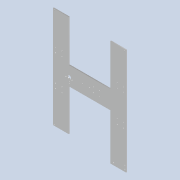
# Autodesk Inventor part: 0008-10-018 Suport Heated Bed
Saved by Autodesk Inventor 2020 (Build 240168000, 168)
## iProperties
Created: 2021-02-27
Part Number: 0008-10-018 Suport Heated Bed
Material: Aluminum 6061
Document SubType Name: Modeling
Designer: Iulian Bors
Density: 2.7 g/cm^3
Appearance: Aluminum - Flat
Mass: 812.917 g
Surface Area: 1617.85 cm^2
Volume: 301.08 cm^3
Description: SUport Pat
Author: Iulian Bors
Subject: 018
Autodesk Inventor part; units mm, degrees
ref_plane "YZ Plane" through (0, 0, 0) normal (1, 0, 0) x (0, 1, 0)
ref_plane "XZ Plane" through (0, 0, 0) normal (0, 1, 0) x (-1, 0, 0)
ref_plane "XY Plane" through (0, 0, 0) normal (0, 0, 1) x (1, 0, 0)
sketch "Sketch1" plane through (0, 0, 0) normal (0, 0, 1) x (1, 0, 0)
  line L0 (-158.5, 220) -> (158.5, 220)
  line L1 (158.5, 220) -> (158.5, -220)
  line L2 (158.5, -220) -> (-158.5, -220)
  line L3 (-158.5, -220) -> (-158.5, 220)
  line L4 (-153.5, 215) -> (153.5, 215) construction
  line L5 (153.5, 215) -> (153.5, -215) construction
  line L6 (153.5, -215) -> (-153.5, -215) construction
  line L7 (-153.5, -215) -> (-153.5, 215) construction
  circle A0 centre (-153.5, 215) radius 2
  circle A1 centre (153.5, 215) radius 2
  circle A2 centre (153.5, -215) radius 2
  circle A3 centre (-153.5, -215) radius 2
  point P0 (0, 0)
  point P1 (0, 220)
  point P2 (-158.5, 0)
  point P3 (0, 215)
  point P4 (-153.5, 0)
  dimension "d0" = 440
  dimension "d1" = 317
  dimension "d3" = 5
  dimension "d4" = 5
  dimension "d5" = 4
  constraints: 16 end point, 4 centre point, 4 coincident, 4 midpoint, 4 parallel, 3 equal radius, 2 horizontal, 2 horizontal alignment, 2 perpendicular, 2 vertical alignment
  measures "d0" distance of L2.end L0.start
  measures "d1" distance of L1.end L2.end
  measures "d3" distance between parallel lines of L3 L7
  measures "d4" distance between parallel lines of L0 L4
  measures "d5" diameter of A0
extrude "Extrusion1" add sketch "Sketch1" along normal blind 4
sketch "Sketch3" plane through (0, 0, 0) normal (0, 0, -1) x (-1, 0, 0)
  line L0 (90, -220) -> (-90, -220)
  line L1 (-90, -220) -> (-90, 220)
  line L2 (-90, 220) -> (90, 220)
  line L3 (90, 220) -> (90, -220)
  line L4 (158.5, -220) -> (-158.5, -220) projected
  line L5 (-158.5, 220) -> (158.5, 220) projected
  line L6 (90, -40) -> (-90, -40)
  line L7 (-90, -40) -> (-90, 40)
  line L8 (-90, 40) -> (90, 40)
  line L9 (90, 40) -> (90, -40)
  point P0 (0, 0)
  point P1 (0, -220)
  point P2 (-90, 0)
  dimension "d11" = 180
  dimension "d12" = 80
  constraints: 16 end point, 4 collinear, 4 parallel, 2 horizontal, 2 midpoint, 2 perpendicular, 1 horizontal alignment, 1 vertical alignment
  measures "d11" distance between parallel lines of L1 L3
  measures "d12" distance between parallel lines of L8 L6
extrude "Extrusion3" cut sketch "Sketch3" against normal through all contours L0 L1 L6 L3 | L8 L1 L2 L3
sketch "Sketch5" plane through (0, 0, 4) normal (0, 0, 1) x (1, 0, 0)
  line L0 (158.5, -240) -> (90, -240)
  line L1 (90, -240) -> (90, -220)
  line L2 (90, -220) -> (158.5, -220)
  line L3 (158.5, -220) -> (158.5, -240)
  line L4 (158.5, 220) -> (90, 220) projected
  line L5 (158.5, -220) -> (158.5, 220) projected
  line L6 (90, 220) -> (90, 40) projected
  circle A0 centre (153.5, -230) radius 2.5
  circle A1 centre (103.5, -230) radius 2.5
  line L7 (90, -220) -> (158.5, -220) projected
  point P0 (0, 0)
  point P1 (124.25, 201.6144)
  point P2 (124.25, -240)
  point P3 (90, -230)
  dimension "d21" = 20
  dimension "d22" = 5
  dimension "d24" = 50
  dimension "d34" = 5
  constraints: 8 end point, 3 collinear, 2 centre point, 2 horizontal alignment, 2 midpoint, 2 parallel, 1 equal radius, 1 horizontal, 1 perpendicular, 1 vertical alignment
  measures "d21" distance of L2.end L0.start
  measures "d22" diameter of A0
  measures "d24" distance of A1.centre A0.centre
  measures "d34" distance from line of A0.centre L3
extrude "Extrusion5" add sketch "Sketch5" against normal up to surface (4 mm away)
sketch "Sketch6" plane through (0, 0, 0) normal (0, 0, -1) x (-1, 0, 0)
  circle A0 centre (119.5, -78) radius 2.1
  circle A1 centre (147.5, -78) radius 2.1
  circle A2 centre (119.5, -57) radius 2.1
  circle A3 centre (147.5, -57) radius 2.1
  line L0 (152.5, -85) -> (142.5, -85)
  line L1 (142.5, -85) -> (142.5, -50)
  line L2 (142.5, -50) -> (152.5, -50)
  line L3 (152.5, -50) -> (152.5, -85)
  line L4 (137.5, -85) -> (129.5, -85)
  line L5 (129.5, -85) -> (129.5, -50)
  line L6 (129.5, -50) -> (137.5, -50)
  line L7 (137.5, -50) -> (137.5, -85)
  line L8 (124.5, -85) -> (114.5, -85)
  line L9 (114.5, -85) -> (114.5, -50)
  line L10 (114.5, -50) -> (124.5, -50)
  line L11 (124.5, -50) -> (124.5, -85)
  circle A4 centre (119.5, 57) radius 2.1
  circle A5 centre (147.5, 57) radius 2.1
  circle A6 centre (119.5, 78) radius 2.1
  circle A7 centre (147.5, 78) radius 2.1
  line L12 (152.5, 50) -> (142.5, 50)
  line L13 (142.5, 50) -> (142.5, 85)
  line L14 (142.5, 85) -> (152.5, 85)
  line L15 (152.5, 85) -> (152.5, 50)
  line L16 (137.5, 50) -> (129.5, 50)
  line L17 (129.5, 50) -> (129.5, 85)
  line L18 (129.5, 85) -> (137.5, 85)
  line L19 (137.5, 85) -> (137.5, 50)
  line L20 (124.5, 50) -> (114.5, 50)
  line L21 (114.5, 50) -> (114.5, 85)
  line L22 (114.5, 85) -> (124.5, 85)
  line L23 (124.5, 85) -> (124.5, 50)
  circle A8 centre (1, 0) radius 2.5
  circle A9 centre (30, 0) radius 2.5
  line L24 (10.5, -12) -> (30.5, -12)
  line L25 (30.5, -12) -> (30.5, -5)
  line L26 (30.5, -5) -> (10.5, -5)
  line L27 (10.5, -5) -> (10.5, -12)
  line L28 (-50, -15.5) -> (40, -15.5)
  line L29 (40, 15.5) -> (40, -15.5)
  line L30 (40, 15.5) -> (-50, 15.5)
  line L31 (-50, -15.5) -> (-50, 15.5)
  line L32 (30.5, 12) -> (10.5, 12)
  line L33 (10.5, 12) -> (10.5, 5)
  line L34 (10.5, 5) -> (30.5, 5)
  line L35 (30.5, 5) -> (30.5, 12)
  circle A10 centre (-16, -10.5) radius 3
  circle A11 centre (-44, -10.5) radius 3
  circle A12 centre (-44, 10.5) radius 3
  circle A13 centre (-16, 10.5) radius 3
  circle A14 centre (-119.5, -57) radius 2.1
  circle A15 centre (-147.5, -57) radius 2.1
  circle A16 centre (-119.5, -78) radius 2.1
  circle A17 centre (-147.5, -78) radius 2.1
  line L36 (-152.5, -50) -> (-142.5, -50)
  line L37 (-142.5, -50) -> (-142.5, -85)
  line L38 (-142.5, -85) -> (-152.5, -85)
  line L39 (-152.5, -85) -> (-152.5, -50)
  line L40 (-137.5, -50) -> (-129.5, -50)
  line L41 (-129.5, -50) -> (-129.5, -85)
  line L42 (-129.5, -85) -> (-137.5, -85)
  line L43 (-137.5, -85) -> (-137.5, -50)
  line L44 (-124.5, -50) -> (-114.5, -50)
  line L45 (-114.5, -50) -> (-114.5, -85)
  line L46 (-114.5, -85) -> (-124.5, -85)
  line L47 (-124.5, -85) -> (-124.5, -50)
  circle A18 centre (-147.5, 57) radius 2.1
  circle A19 centre (-119.5, 57) radius 2.1
  circle A20 centre (-147.5, 78) radius 2.1
  circle A21 centre (-119.5, 78) radius 2.1
  line L48 (-114.5, 50) -> (-124.5, 50)
  line L49 (-124.5, 50) -> (-124.5, 85)
  line L50 (-124.5, 85) -> (-114.5, 85)
  line L51 (-114.5, 85) -> (-114.5, 50)
  line L52 (-129.5, 50) -> (-137.5, 50)
  line L53 (-137.5, 50) -> (-137.5, 85)
  line L54 (-137.5, 85) -> (-129.5, 85)
  line L55 (-129.5, 85) -> (-129.5, 50)
  line L56 (-142.5, 50) -> (-152.5, 50)
  line L57 (-152.5, 50) -> (-152.5, 85)
  line L58 (-152.5, 85) -> (-142.5, 85)
  line L59 (-142.5, 85) -> (-142.5, 50)
  point P0 (0, 0)
  constraints: 120 end point, 30 horizontal, 30 vertical, 22 centre point, 104 other
hole "Hole1" at (-147.5, -78, 0) at (-119.5, -78, 0) at (-119.5, -57, 0) at (-147.5, -57, 0) at (-30, 0, 0) at (0, 0, 0) at (16, -10.5, 0) at (44, -10.5, 0) at (44, 10.5, 0) at (16, 10.5, 0) at (-119.5, 57, 0) at (-119.5, 78, 0) at (-147.5, 78, 0) at (-147.5, 57, 0) at (119.5, 57, 0) at (147.5, 57, 0) at (147.5, 78, 0) at (119.5, 78, 0) at (147.5, -78, 0) at (119.5, -78, 0) at (119.5, -57, 0) at (147.5, -57, 0) direction (0, 0, 1) diameter 5 end through all
sketch "Sketch7" plane through (0, 0, 0) normal (0, 0, -1) x (-1, 0, 0)
  line L0 (-60, -15.1293) -> (-60, -45.1293)
  line L1 (-71, -45.1293) -> (-60, -45.1293)
  line L2 (-71, -45.1293) -> (-71, -15.1293)
  line L3 (-71, -15.1293) -> (-60, -15.1293)
  circle A0 centre (88, -28) radius 2
  circle A1 centre (88, -20) radius 2
  line L4 (-90, -40) -> (90, -40) projected
  circle A2 centre (88, -5) radius 7.5
  circle A3 centre (76, -10) radius 3
  circle A4 centre (103, -10) radius 3
  line L5 (84.5, -12.7391) -> (91.5, -12.7391) projected
  line L6 (84.5, -12.7391) -> (84.5, -22.7391) projected
  line L7 (93.5, -12.7391) -> (93.5, -22.7391) projected
  line L8 (-107, -6) -> (107, -6) projected
  line L9 (-107, -220) -> (-107, -6) projected
  line L10 (107, -220) -> (-107, -220) projected
  line L11 (107, -6) -> (107, -220) projected
  circle A5 centre (104.5, -217.5) radius 1.5 projected
  circle A6 centre (-104.5, -217.5) radius 1.5 projected
  circle A7 centre (-104.5, -8.5) radius 1.5 projected
  circle A8 centre (104.5, -8.5) radius 1.5 projected
  point P0 (0, 0)
  dimension "d35" = 4
  dimension "d37" = 8
  dimension "d38" = 12
  dimension "d39" = 15
  dimension "d40" = 35
  dimension "d41" = 6
  dimension "d42" = 12
  dimension "d43" = 15
  dimension "d44" = 5
  dimension "d47" = 5.5
  constraints: 8 end point, 5 centre point, 2 equal radius, 2 horizontal, 2 vertical, 2 vertical alignment, 1 horizontal alignment, 4 other
  measures "d35" diameter of A0
  measures "d37" distance of A1.centre A0.centre
  measures "d38" distance from line of L4 A0.centre
  measures "d39" diameter of A2
  measures "d40" distance from line of A2.centre L4
  measures "d41" diameter of A3
  measures "d42" horizontal distance of A2.centre A3.centre
  measures "d43" horizontal distance of A2.centre A4.centre
  measures "d44" vertical distance of A3.centre A2.centre
  measures "d47" distance from line of L7 A0.centre
extrude "Extrusion6" cut sketch "Sketch7" against normal through all contours A0 | A1 | A2 L8 | L8 A2 | A3 | A4 A8 | A8 A4 picked at (101.8731, -11.3773) picked at (104.2239, -7.9666)
equation "\"d43\" = d39"
body "Solid1"
